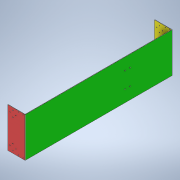
# Autodesk Inventor part: Caja - Base
Saved by Autodesk Inventor 2021 (Build 250183000, 183)
## iProperties
Created: 2022-01-22
Part Number: Caja - Base
Material: Generic
Document SubType Name: Modeling
Designer: deuts
Density: 1 g/cm^3
Appearance: Default
Author: deuts
Autodesk Inventor part; units mm, degrees
ref_plane "YZ Plane" through (0, 0, 0) normal (1, 0, 0) x (0, 1, 0)
ref_plane "XZ Plane" through (0, 0, 0) normal (0, 1, 0) x (-1, 0, 0)
ref_plane "XY Plane" through (0, 0, 0) normal (0, 0, 1) x (1, 0, 0)
sketch "Sketch1" plane through (0, 0, 0) normal (0, 1, 0) x (-1, 0, 0)
  line L0 (1, 0) -> (70.5, 0)
  line L1 (0, -1) -> (0, -593)
  line L2 (1, -594) -> (70.5, -594)
  line L3 (70.5, -1.6) -> (2.6, -1.6)
  line L4 (1.6, -2.6) -> (1.6, -591.4)
  line L5 (2.6, -592.4) -> (70.5, -592.4)
  line L6 (70.5, 0) -> (70.5, -1.6)
  line L7 (70.5, -592.4) -> (70.5, -594)
  arc A0 (1, 0) -> (0, -1) centre (1, -1) ccw
  arc A1 (0, -593) -> (1, -594) centre (1, -593) ccw
  arc A2 (2.6, -1.6) -> (1.6, -2.6) centre (2.6, -2.6) ccw
  arc A3 (1.6, -591.4) -> (2.6, -592.4) centre (2.6, -591.4) ccw
  point P0 (0, 0)
  point P1 (0, -594)
  dimension "d0" = 70.5
  dimension "d1" = 594
  dimension "d2" = 70.5
  dimension "d3" = 1.6
  dimension "d4" = 1
  dimension "d5" = 1
  constraints: 16 end point, 8 point on circle, 8 tangent, 4 centre point, 4 point on line, 2 equal radius, 2 perpendicular, 2 vertical, 1 collinear, 1 horizontal, 2 other
  measures "d0" distance of point (0, 0) L0.end
  measures "d1" distance of point (0, 0) point (0, -594)
  measures "d2" distance of point (0, -594) L2.end
  measures "d3" distance between parallel lines of L0 L3
  measures "d4" radius of A0
  measures "d5" radius of A1
extrude "Extrusion1" add sketch "Sketch1" along normal mid plane 160
sketch "Sketch2" plane through (-70.5, -80, 0) normal (0, 0, 1) x (1, 0, 0)
  line L0 (0, 0) -> (0, 160) projected
  line L1 (67.9, 160) -> (0, 160) projected
  line L2 (0, 0) -> (67.9, 0) projected
  circle A0 centre (20.9, 10) radius 1.75
  circle A1 centre (8.9, 22) radius 1.75
  circle A2 centre (20.9, 34) radius 1.75
  circle A3 centre (32.9, 22) radius 1.75
  line L3 (70.5, 80) -> (70.5, 160) projected
  constraints: 4 centre point
hole "Hole1" at (-49.6, -70, 0) at (-37.6, -58, 0) at (-49.6, -46, 0) at (-61.6, -58, 0) direction (0, 0, -1) diameter 3 end through all
mirror "Mirror1" about plane through (0, 0, 0) normal (0, 1, 0) of "Hole1"
sketch "Sketch3" plane through (-1.6, -80, -2.6) normal (-1, 0, 0) x (0, 0, 1)
  line L0 (-589.8, 0) -> (-589.8, 160) projected
  line L1 (-588.8, 160) -> (0, 160) projected
  line L2 (0, 0) -> (-588.8, 0) projected
  line L3 (-588.8, 0) -> (-588.8, 160) projected
  circle A0 centre (-420.4, 112.5) radius 2
  circle A1 centre (-400.4, 112.5) radius 2
  point P0 (2.6, 80)
  dimension "d28" = 4
  dimension "d30" = 4
  dimension "d33" = 47.5
  dimension "d35" = 20
  constraints: 2 centre point
  measures "d28" diameter of A0
  measures "d30" diameter of A1
  measures "d33" distance from line of L1 A0.centre
  measures "d35" distance of A1.centre A0.centre
extrude "Extrusion2" cut sketch "Sketch3" against normal blind 3
mirror "Mirror2" about plane through (0, 0, 0) normal (0, 1, 0) of "Extrusion2"
sketch "Sketch4" plane through (-1, 80, -594) normal (0, 0, -1) x (-1, 0, 0)
  line L0 (69.5, 0) -> (1.6, 0) projected
  line L1 (1.6, 0) -> (8.6, 0)
  circle A0 centre (7.61, -4.6) radius 2
  circle A1 centre (25.61, -4.6) radius 2
  line L2 (0, -160) -> (0, 0) projected
  line L3 (69.5, -160) -> (69.5, 0) projected
  point P0 (-1, -80)
  dimension "d38" = 4
  dimension "d40" = 4
  dimension "d48" = 4.6
  dimension "d49" = 4.6
  dimension "d51" = 18
  dimension "d52" = 43.89
  constraints: 2 centre point, 2 end point, 1 point on line
  measures "d38" diameter of A0
  measures "d40" diameter of A1
  measures "d48" distance from line of L0 A0.centre
  measures "d49" distance from line of L0 A1.centre
  measures "d51" distance of A1.centre A0.centre
  measures "d52" distance from line of L3 A1.centre
hole "Hole2" at (-26.61, 75.4, -594) at (-8.61, 75.4, -594) direction (0, 0, 1) diameter 3 end through all
mirror "Mirror3" about plane through (0, 0, 0) normal (0, 1, 0) of "Hole2"
body "Solid1"
